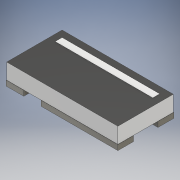
# Autodesk Inventor part: 23-5m00
Saved by Autodesk Inventor 2018 (Build 220112000, 112)
## iProperties
Created: 2019-09-30
Part Number: 23-5m00
Material: Copper
Document SubType Name: Modeling
Designer: Bradley
Density: 8.94 g/cm^3
Appearance: Smooth - White
Author: Bradley
Autodesk Inventor part; units mm, degrees
ref_plane "YZ Plane" through (0, 0, 0) normal (1, 0, 0) x (0, 1, 0)
ref_plane "XZ Plane" through (0, 0, 0) normal (0, 1, 0) x (-1, 0, 0)
ref_plane "XY Plane" through (0, 0, 0) normal (0, 0, 1) x (1, 0, 0)
sketch "Sketch1" plane through (0, 0, 0) normal (0, 0, 1) x (1, 0, 0)
  line L0 (-1.6, 0.8) -> (-1.1, 0.8)
  line L1 (-1.1, 0.8) -> (-1.1, 0.35)
  line L2 (-1.1, 0.35) -> (-1.6, 0.35)
  line L3 (-1.6, 0.35) -> (-1.6, 0.8)
  line L4 (-1.6, -0.35) -> (-1.1, -0.35)
  line L5 (-1.1, -0.35) -> (-1.1, -0.8)
  line L6 (-1.1, -0.8) -> (-1.6, -0.8)
  line L7 (-1.6, -0.8) -> (-1.6, -0.35)
  line L8 (-0.6, 0.8) -> (1.6, 0.8)
  line L9 (1.6, 0.8) -> (1.6, 0.35)
  line L10 (1.6, 0.35) -> (-0.6, 0.35)
  line L11 (-0.6, 0.35) -> (-0.6, 0.8)
  line L12 (-0.6, -0.35) -> (1.6, -0.35)
  line L13 (1.6, -0.35) -> (1.6, -0.8)
  line L14 (1.6, -0.8) -> (-0.6, -0.8)
  line L15 (-0.6, -0.8) -> (-0.6, -0.35)
  line L16 (-1.6, 0.8) -> (1.6, 0.8)
  line L17 (1.6, 0.8) -> (1.6, -0.8)
  line L18 (1.6, -0.8) -> (-1.6, -0.8)
  line L19 (-1.6, -0.8) -> (-1.6, 0.8)
  line L20 (1.595, 0.795) -> (-1.595, 0.795)
  line L21 (-1.595, 0.795) -> (-1.595, -0.795)
  line L22 (-1.595, -0.795) -> (1.595, -0.795)
  line L23 (1.595, -0.795) -> (1.595, 0.795)
  point P0 (0, 0)
  point P1 (0, 0.8)
  point P2 (-1.6, 0)
  dimension "d0" = 2.2
  dimension "d1" = 0.45
  dimension "d2" = 0.7
  dimension "d3" = 0.5
  dimension "d4" = 0.5
  dimension "d7" = 0.005
  constraints: 48 end point, 12 parallel, 8 point on line, 6 perpendicular, 5 horizontal, 2 midpoint, 1 collinear, 1 horizontal alignment, 1 vertical alignment, 3 other
  measures "d0" distance of L8.start L8.end
  measures "d1" distance of L8.end L9.end
  measures "d2" distance between parallel lines of L12 L10
  measures "d3" distance between parallel lines of L1 L11
  measures "d4" distance of L0.start L0.end
  measures "d7" distance between parallel lines of L16 L20
extrude "Extrusion1" add sketch "Sketch1" against normal blind 0.15 contours L0 L1 L20 L21 L2 L3 | L1 L2 L21 L20 | L8 L9 L10 L23 L20 L11 | L4 L21 L22 L5 L6 L7 | L20 L23 L10 L11 | L4 L5 L22 L21 | L13 L14 L15 L22 L23 L12 | L23 L22 L15 L12
extrude "Extrusion2" add sketch "Sketch1" along normal blind 0.45 contours L20 L11 L10 L23 L12 L15 L22 L5 L4 L21 L2 L1 | L1 L2 L21 L20 | L20 L23 L10 L11 | L4 L5 L22 L21 | L23 L22 L15 L12
sketch "Sketch2" plane through (0, 0, 0.45) normal (0, 0, 1) x (1, 0, 0)
  line L0 (1.595, 0.795) -> (-1.595, 0.795) projected
  line L1 (-1.595, 0.795) -> (-1.595, -0.795) projected
  line L2 (-1.595, -0.795) -> (1.595, -0.795) projected
  line L3 (1.595, -0.795) -> (1.595, 0.795) projected
  line L4 (-1.4, 0.6) -> (1.4, 0.6)
  line L5 (1.4, 0.6) -> (1.4, 0.4)
  line L6 (1.4, 0.4) -> (-1.4, 0.4)
  line L7 (-1.4, 0.4) -> (-1.4, 0.6)
  point P0 (0, 0)
  point P1 (0, 0.4)
  dimension "d10" = 2.8
  dimension "d11" = 0.2
  dimension "d12" = 0.4
  constraints: 8 end point, 2 parallel, 1 horizontal, 1 midpoint, 1 perpendicular, 1 vertical alignment
  measures "d10" distance of L5.end L6.end
  measures "d11" distance of L4.end L5.end
  measures "d12" distance from line of point (0, 0) L6
extrude "Extrusion3" add sketch "Sketch2" along normal blind 0.01 contours L4 L5 L6 L7
body "Solid1"
